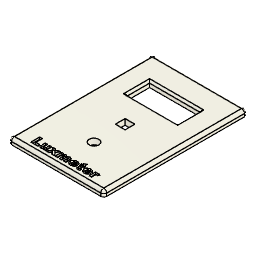
Luxmeter_Cover (Autodesk Fusion 360 design; units mm, degrees)
Autodesk Fusion 360 part; units mm, degrees
note: some values were not read from the file. Set by a fixed rule: which sketch regions a step uses.
sketch "Sketch1" plane through (0, 0, 0) normal (0, 0, 1) x (1, 0, 0)
  line L0 (0, 0) -> (49, 0)
  line L1 (49, 0) -> (49, 74)
  line L2 (49, 74) -> (0, 74)
  line L3 (0, 74) -> (0, 0)
  dimension "d1" = 74
  dimension "d2" = 49
  constraint horizontal L0
  constraint vertical L1
  constraint horizontal L2
  constraint vertical L3
  constraint coincident L0.start L3.end
  measures "d1" distance of L0.start L2.end
  measures "d2" distance of L0.start L0.end
extrude "Extrude1" add sketch "Sketch1" along normal blind 5
sketch "Sketch2" plane through (0, 0, 5) normal (0, 0, 1) x (-1, 0, 0)
  line L0 (0, -74) -> (0, 0)
  line L1 (0, 0) -> (-49, 0)
  line L2 (-49, 0) -> (-49, -74)
  line L3 (-49, -74) -> (0, -74)
  circle A0 centre (-24.4735, -19.513) radius 2.5
  line L4 (-21.9948, -33) -> (-21.9948, -38)
  line L5 (-21.9948, -38) -> (-26.9948, -38)
  line L6 (-26.9948, -38) -> (-26.9948, -33)
  line L7 (-26.9948, -33) -> (-21.9948, -33)
  line L8 (-11.4974, -49.6) -> (-11.4974, -61.1)
  line L9 (-11.4974, -61.1) -> (-37.4974, -61.1)
  line L10 (-37.4974, -61.1) -> (-37.4974, -49.6)
  line L11 (-37.4974, -49.6) -> (-11.4974, -49.6)
  line L12 (-37.4974, -49.6) -> (-11.4974, -61.1) construction
  line L13 (-11.4974, -49.6) -> (-37.4974, -61.1) construction
  line L14 (-24.5, -74) -> (-24.5, 0)
  dimension "d5" = 26
  dimension "d6" = 11.5
  dimension "d7" = 11.6
  dimension "d8" = 13.487
  constraint horizontal L11
  constraint perpendicular L8 L11
  constraint parallel L9 L11
  constraint parallel L8 L10
  constraint midpoint L3 L14.start
  constraint midpoint L1 L14.end
  measures "d5" distance of L9.end L8.end
  measures "d6" distance of L8.start L8.end
  measures "d7" distance of L5 L11
  measures "d8" distance of A0.centre L7
extrude "Extrude2" cut sketch "Sketch2" against normal blind 5 contours L8 L9 L11 L14 | L9 L10 L11 L14 | A0 L14 | A0 L14 | L4 L5 L7 L14 | L5 L6 L7 L14
fillet "Fillet1" radius 1 4 edges at (24.4974, 61.1, 5) (37.4974, 55.35, 5) (11.4974, 55.35, 5) (24.4974, 49.6, 5)
sketch "Sketch4" plane through (0, 0, 0) normal (0, 0, -1) x (1, 0, 0)
  line L0 (37.4974, -61.1) -> (11.4974, -61.1)
  line L1 (11.4974, -61.1) -> (11.4974, -49.6)
  line L2 (11.4974, -49.6) -> (37.4974, -49.6)
  line L3 (37.4974, -49.6) -> (37.4974, -61.1)
  line L4 (26.9948, -38) -> (21.9948, -38)
  line L5 (21.9948, -38) -> (21.9948, -33)
  line L6 (21.9948, -33) -> (26.9948, -33)
  line L7 (26.9948, -33) -> (26.9948, -38)
  circle A0 centre (24.4735, -19.513) radius 2.5
  line L8 (0, 0) -> (0, -74)
  line L9 (0, -74) -> (49, -74)
  line L10 (49, -74) -> (49, 0)
  line L11 (49, 0) -> (0, 0)
  line L12 (49, -74) -> (49, 0)
  line L13 (49, 0) -> (0, 0)
  line L14 (0, 0) -> (0, -74)
  line L15 (0, -74) -> (49, -74)
  line L16 (2.75, -71.25) -> (46.25, -71.25)
  line L17 (46.25, -71.25) -> (46.25, -2.75)
  line L18 (46.25, -2.75) -> (2.75, -2.75)
  line L19 (2.75, -2.75) -> (2.75, -71.25)
  dimension "d22" = 0
  dimension "d23" = -2.75
  measures "d22" distance of L11
extrude "Extrude4" cut sketch "Sketch4" against normal blind 2 contours L8 L9 L10 L11 L12 L13 L14 L15
fillet "Fillet3" radius 1.5 8 edges at (49, 74, 3.5) (0, 74, 3.5) (0, 0, 3.5) (49, 0, 3.5) (24.5, 74, 5) (49, 37, 5) (24.5, 0, 5) (0, 37, 5)
sketch "Sketch5" plane through (0, 0, 0) normal (0, 0, -1) x (1, 0, 0)
  line L0 (46.25, -2.75) -> (2.75, -2.75)
  line L1 (2.75, -2.75) -> (2.75, -71.25)
  line L2 (2.75, -71.25) -> (46.25, -71.25)
  line L3 (46.25, -71.25) -> (46.25, -2.75)
  line L4 (37.4974, -61.1) -> (11.4974, -61.1)
  line L5 (11.4974, -61.1) -> (11.4974, -49.6)
  line L6 (11.4974, -49.6) -> (37.4974, -49.6)
  line L7 (37.4974, -49.6) -> (37.4974, -61.1)
  line L8 (26.9948, -38) -> (21.9948, -38)
  line L9 (21.9948, -38) -> (21.9948, -33)
  line L10 (21.9948, -33) -> (26.9948, -33)
  line L11 (26.9948, -33) -> (26.9948, -38)
  circle A0 centre (24.4735, -19.513) radius 2.5
  line L12 (2.75, -71.25) -> (46.25, -71.25)
  line L13 (46.25, -71.25) -> (46.25, -2.75)
  line L14 (46.25, -2.75) -> (2.75, -2.75)
  line L15 (2.75, -2.75) -> (2.75, -71.25)
  line L16 (4.75, -69.25) -> (44.25, -69.25)
  line L17 (44.25, -69.25) -> (44.25, -4.75)
  line L18 (44.25, -4.75) -> (4.75, -4.75)
  line L19 (4.75, -4.75) -> (4.75, -69.25)
  dimension "d28" = 0
  dimension "d29" = -2
  measures "d28" distance of L0
extrude "Extrude5" cut sketch "Sketch5" against normal blind 2 contours L16 L17 L18 L19
extrude "Extrude6" cut 1 faces at (3.4167, 47.75, 0) along direction (0, 0, 1) blind 0.1
sketch "Sketch6" plane through (0, 0, 5) normal (0, 0, 1) x (-1, 0, 0)
  line L0 (-10.4974, -62.1) -> (-38.4974, -62.1)
  line L1 (-38.4974, -62.1) -> (-38.4974, -48.6)
  line L2 (-38.4974, -48.6) -> (-10.4974, -48.6)
  line L3 (-10.4974, -48.6) -> (-10.4974, -62.1)
  line L4 (-21.9948, -38) -> (-26.9948, -38)
  line L5 (-26.9948, -38) -> (-26.9948, -33)
  line L6 (-26.9948, -33) -> (-21.9948, -33)
  line L7 (-21.9948, -33) -> (-21.9948, -38)
  circle A0 centre (-24.4735, -19.513) radius 2.5
  line L8 (-1.5, -72.5) -> (-1.5, -1.5)
  line L9 (-1.5, -1.5) -> (-47.5, -1.5)
  line L10 (-47.5, -1.5) -> (-47.5, -72.5)
  line L11 (-47.5, -72.5) -> (-1.5, -72.5)
  line L12 (-1.5, -1.5) -> (-47.5, -1.5) construction
  line L13 (-47.5, -1.5) -> (-47.5, -9.5) construction
  line L14 (-47.5, -9.5) -> (-1.5, -9.5) construction
  line L15 (-1.5, -9.5) -> (-1.5, -1.5) construction
  dimension "d34" = 4.5
  dimension "d36" = 8
  text T0 "Luxmeter" font "Arial Black" height 4.5 align centre middle in box 46 x 8 at (-1.5, -1.5) x (-1, 0) y (0, -1) spacing 1
  constraint coincident L10
  constraint coincident L8.end
extrude "Extrude7" cut sketch "Sketch6" against normal blind 1 text T0
fillet "Fillet2" [suppressed]
equation "d35 = 'Luxmeter'"
